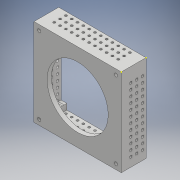
# Autodesk Inventor part: Middle
Saved by Autodesk Inventor 2018 (Build 220112000, 112)
## iProperties
Created: 2018-04-09
Part Number: Middle
Material: Generic
Document SubType Name: Modeling
Designer: a
Density: 1 g/cm^3
Appearance: Default
Author: a
## iProperties of the stored document Part1_3DPrint.ipt
Created: 2018-04-09
Part Number: Part1_3DPrint
Material: Generic
Document SubType Name: Modeling
Designer: a
Density: 1 g/cm^3
Appearance: Default
Author: a
Autodesk Inventor part; units mm, degrees
ref_plane "YZ Plane" through (0, 0, 0) normal (1, 0, 0) x (0, 1, 0)
ref_plane "XZ Plane" through (0, 0, 0) normal (0, 1, 0) x (-1, 0, 0)
ref_plane "XY Plane" through (0, 0, 0) normal (0, 0, 1) x (1, 0, 0)
sketch "Sketch1" plane through (0, 0, 0) normal (0, 1, 0) x (-1, 0, 0)
  point P0 (0, 0)
sketch "Sketch2" plane through (0, 0, 0) normal (0, 1, 0) x (-1, 0, 0)
  line L0 (0, 0) -> (150, 0)
  line L1 (150, 0) -> (150, -150)
  line L2 (150, -150) -> (0, -150)
  line L3 (0, -150) -> (0, 0)
  dimension "d0" = 150
  dimension "d1" = 150
  constraints: 8 end point, 2 parallel, 1 horizontal, 1 perpendicular
  measures "d0" distance of L1.end L2.end
  measures "d1" distance of L0.end L1.end
extrude "Extrusion1" add sketch "Sketch2" along normal blind 7.5
sketch "Sketch3" plane through (0, 7.5, 0) normal (0, 1, 0) x (1, 0, 0)
  line L0 (-150, 150) -> (-150, 0) projected
  circle A0 centre (-75, 75) radius 52.5
  point P0 (0, 0)
  constraints: 1 centre point
extrude "Extrusion2" cut sketch "Sketch3" against normal blind 7.5
sketch "Sketch4" plane through (0, 7.5, 0) normal (0, 1, 0) x (1, 0, 0)
  line L0 (0, 0) -> (-150, 0) projected
  line L1 (0, 150) -> (0, 0) projected
  line L2 (-150, 0) -> (0, 0)
  line L3 (0, 0) -> (0, 150)
  line L4 (0, 150) -> (-150, 150)
  line L5 (-150, 150) -> (-150, 0)
  line L6 (-146, 4) -> (-4, 4)
  line L7 (-4, 4) -> (-4, 146)
  line L8 (-4, 146) -> (-146, 146)
  line L9 (-146, 146) -> (-146, 4)
  dimension "d7" = 4
  constraints: 16 end point, 4 parallel, 2 perpendicular, 1 horizontal, 3 other
  measures "d7" distance between parallel lines of L5 L9
extrude "Extrusion3" add sketch "Sketch4" along normal blind 35
sketch "Sketch5" plane through (0, 7.5, 0) normal (0, 1, 0) x (1, 0, 0)
  line L0 (-146, 146) -> (-146, 4) projected
  line L1 (-146, 4) -> (-136, 4)
  line L2 (-136, 4) -> (-136, 14)
  line L3 (-136, 14) -> (-146, 14)
  line L4 (-146, 14) -> (-146, 4)
  point P0 (0, 0)
  dimension "d10" = 10
  dimension "d11" = 10
  constraints: 8 end point, 2 parallel, 1 horizontal, 1 perpendicular
  measures "d10" distance of L3.end L2.end
  measures "d11" distance of L2.end L1.end
extrude "Extrusion4" add sketch "Sketch5" along normal blind 35
pattern_linear "Rectangular Pattern1" count 2 spacing 132 along (0, 0, -1) count 2 spacing 132 along (1, 0, 0) of "Extrusion4"
sketch "Sketch6" plane through (0, 42.5, 0) normal (0, 1, 0) x (1, 0, 0)
  line L0 (-136, 14) -> (-146, 14) projected
  line L1 (-141, 14) -> (-141, 0)
  line L2 (0, 0) -> (-150, 0) projected
  circle A0 centre (-141, 9) radius 2.75
  dimension "d20" = 5.5
  constraints: 2 end point, 2 point on line, 1 centre point, 1 midpoint, 1 vertical
  measures "d20" diameter of A0
extrude "Extrusion5" cut sketch "Sketch6" against normal blind 80
pattern_linear "Rectangular Pattern2" count 2 spacing 132 along (0, 0, -1) count 2 spacing 132 along (1, 0, 0) of "Extrusion5"
sketch "Sketch7" plane through (0, 0, 0) normal (1, 0, 0) x (0, 0, -1)
  circle A0 centre (24.4072, 36.2876) radius 2.1965
  point P0 (0, 0)
  constraints: 1 centre point
extrude "Extrusion6" cut sketch "Sketch7" against normal blind 300
pattern_linear "Rectangular Pattern3" count 12 spacing 10 along (0, 0, -1) count 3 spacing 10 along (0, -1, 0) of "Extrusion6"
sketch "Sketch8" plane through (0, 0, -150) normal (0, 0, -1) x (-1, 0, 0)
  circle A0 centre (21.3506, 36.1702) radius 1.9726
  point P0 (0, 0)
  constraints: 1 centre point
extrude "Extrusion7" cut sketch "Sketch8" against normal blind 300
pattern_linear "Rectangular Pattern4" count 12 spacing 10 along (-1, 0, 0) count 3 spacing 10 along (0, -1, 0) of "Extrusion7"
sketch "Sketch9" plane through (0, 42.5, 0) normal (0, 1, 0) x (1, 0, 0)
  point P0 (0, 0)
body "Solid1"
